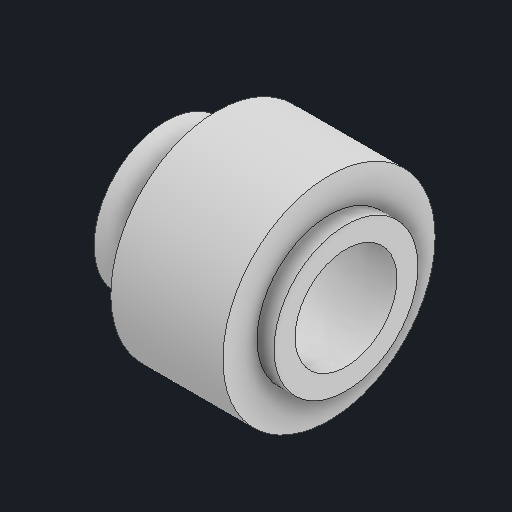
# Autodesk Inventor part: Buge
Saved by Autodesk Inventor 2024 (Build 280153000, 153)
## iProperties
Created: 2022-12-08
Part Number: Buge
Material: Genérico
Document SubType Name: Modeling
Designer: juanj
Density: 1 g/cm^3
Appearance: Valor por defecto
Author: juanj
Autodesk Inventor part; units mm, degrees
ref_plane "YZ Plane" through (0, 0, 0) normal (1, 0, 0) x (0, 1, 0)
ref_plane "XZ Plane" through (0, 0, 0) normal (0, 1, 0) x (-1, 0, 0)
ref_plane "XY Plane" through (0, 0, 0) normal (0, 0, 1) x (1, 0, 0)
sketch "Boceto6" plane through (0, 0, 0) normal (1, 0, 0) x (0, 1, 0)
  circle A0 centre (0, 0) radius 6
  circle A1 centre (0, 0) radius 12.5
  circle A2 centre (0, 0) radius 8.475
  dimension "d16" = 12
  dimension "d17" = 25
  dimension "d18" = 16.95
  constraints: 3 centre point, 3 coincident
  measures "d16" diameter of A0
  measures "d17" diameter of A1
  measures "d18" diameter of A2
extrude "Extrusión6" add sketch "Boceto6" along normal blind 4 and the other way blind 4 contours A1
extrude "Extrusión7" add sketch "Boceto6" along normal blind 6.2 and the other way blind 10 contours A2
sketch "Boceto7" plane through (4, 0, 0) normal (1, 0, 0) x (0, 0, -1)
  circle A0 centre (0, 0) radius 6
  circle A1 centre (0, 0) radius 8.475
  circle A2 centre (0, 0) radius 12.5
  constraints: 3 centre point, 3 coincident
extrude "Extrusión8" add sketch "Boceto7" along normal blind 5.2 contours A2
extrude "Extrusión9" add sketch "Boceto7" along normal blind 7.2 contours A1
